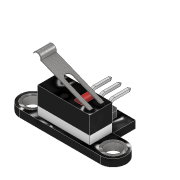
# Autodesk Inventor part: limit_switch
Saved by Autodesk Inventor 2022 (Build 260153000, 153)
## iProperties
Created: 2022-11-16
Part Number: limit_switch
Material: Generic
Document SubType Name: Modeling
Designer: ferna
Density: 1 g/cm^3
Appearance: Default
Author: ferna
Autodesk Inventor part; units mm, degrees
sketch "Sketch1" plane through (0, 0, 0) normal (0, 1, 0) x (-1, 0, 0)
  line L0 (0, 0) -> (14.5, 0)
  line L1 (14.5, 0) -> (14.5, -6)
  line L2 (14.5, -6) -> (0, -6)
  line L3 (0, -6) -> (0, 0)
  line L4 (0, 0) -> (14.5, 0)
  line L5 (14.5, 0) -> (14.5, 7)
  line L6 (14.5, 7) -> (0, 7)
  line L7 (0, 7) -> (0, 0)
  line L8 (14.5, 3.5) -> (18, 3.5)
  line L9 (0, 3.5) -> (-3.5, 3.5)
  circle A0 centre (18, 3.5) radius 3.5
  circle A1 centre (-3.5, 3.5) radius 3.5
  line L10 (18, 7) -> (14.5, 7)
  line L11 (18, 0) -> (14.5, 0)
  line L12 (0, 0) -> (-3.5, 0)
  line L13 (-3.5, 7) -> (0, 7)
  circle A2 centre (18, 3.5) radius 2
  circle A3 centre (-3.5, 3.5) radius 2
  dimension "d0" = 14.5
  dimension "d1" = 6
  dimension "d2" = 7
  dimension "d3" = 3.5
  dimension "d4" = 3.5
  dimension "d5" = 4
  constraints: 28 end point, 6 point on circle, 5 parallel, 4 centre point, 4 coincident, 4 horizontal, 2 midpoint, 2 perpendicular, 2 point on line, 2 tangent
  measures "d0" distance of L1.end L2.end
  measures "d1" distance of L0.end L1.end
  measures "d2" distance of L5.end L4.end
  measures "d3" distance of L8.start L8.end
  measures "d4" distance of L9.start L9.end
  measures "d5" diameter of A2
extrude "Extrusion1" add sketch "Sketch1" along normal blind 2
sketch "Sketch2" plane through (0, 2, 0) normal (0, 1, 0) x (1, 0, 0)
  line L0 (0, 0) -> (0, 6) projected
  line L1 (0, 0) -> (0, -3)
  line L2 (0, -3) -> (-7.25, -3)
  line L3 (-0.25, -6) -> (-14.25, -6)
  line L4 (-14.25, -6) -> (-14.25, 0)
  line L5 (-14.25, 0) -> (-0.25, 0)
  line L6 (-0.25, 0) -> (-0.25, -6)
  line L7 (-0.25, -6) -> (-14.25, 0) construction
  line L8 (-14.25, -6) -> (-0.25, 0) construction
  dimension "d8" = 3
  dimension "d9" = 7.25
  dimension "d10" = 14
  dimension "d11" = 6
  constraints: 16 end point, 2 midpoint, 2 parallel, 2 perpendicular, 1 horizontal, 1 vertical
  measures "d8" distance of L0.start L1.end
  measures "d9" distance of L1.end L2.end
  measures "d10" distance of L4.end L5.end
  measures "d11" distance of L3.end L4.end
extrude "Extrusion2" add sketch "Sketch2" along normal blind 7
ref_plane "Work Plane1" through (-14.25, 2, 5) normal (0, 0, 1) x (1, 0, 0)
sketch "Sketch3" plane through (-14.25, 2, 5) normal (0, 0, 1) x (1, 0, 0)
  line L0 (14, 7) -> (0, 7) projected
  line L1 (12.8898, 7) -> (0, 12.2078)
  line L2 (12.8898, 7) -> (26.7918, 7) construction
  line L3 (0, 12.2078) -> (0, 12.0078)
  line L4 (0, 12.0078) -> (12.3948, 7)
  line L5 (0, 12.0078) -> (13.3682, 12.0078) construction
  line L6 (12.3948, 7) -> (12.8898, 7)
  arc A0 (0, 12.2078) -> (-2.0675, 13.0431) centre (-1.0827, 12.5043) ccw
  line L7 (-2.0675, 13.0431) -> (-2.0675, 12.8431)
  arc A1 (-0.2257, 12.099) -> (-2.0675, 12.8431) centre (-1.1902, 12.3632) ccw
  line L8 (-0.2257, 12.099) -> (0, 12.0078)
  point P0 (14.25, -2)
  point P1 (-0.2257, 12.099)
  dimension "d15" = 158
  dimension "d16" = 0.2
  dimension "d17" = 22
  dimension "d18" = 0.2
  dimension "d19" = 1
  constraints: 16 end point, 4 point on circle, 3 horizontal, 3 point on line, 2 centre point, 2 equal length, 1 perpendicular, 1 vertical
  measures "d15" angle of L2 L1
  measures "d16" distance of L1.end L3.end
  measures "d17" angle of L4 L5
  measures "d18" distance of L7.start L7.end
  measures "d19" radius of A1
extrude "Extrusion3" add sketch "Sketch3" against normal blind 4
sketch "Sketch4" plane through (-18, 0, 7) normal (0, 0, 1) x (1, 0, 0)
  line L0 (0, 2) -> (-3.5, 2) projected
  line L1 (-3.5, 2) -> (26.8199, 2)
  line L2 (26.8199, 2) -> (26.8199, 16.7787)
  line L3 (26.8199, 16.7787) -> (-3.5, 16.7787)
  line L4 (-3.5, 16.7787) -> (-3.5, 2)
  point P0 (18, 0)
  constraints: 8 end point, 2 parallel, 1 horizontal, 1 perpendicular
split body "Split1" sketch "Sketch4" result two bodies curves L4 L1 L2 L3 first body at (-4.9167, 4.3333, 0.5)
sketch "Sketch5" plane through (-14.25, 9, 6) normal (0, 0, 1) x (1, 0, 0)
  line L0 (-3.2734, -4.7413) -> (21.2547, -4.7413)
  line L1 (21.2547, -4.7413) -> (21.2547, 8.151)
  line L2 (21.2547, 8.151) -> (-3.2734, 8.151)
  line L3 (-3.2734, 8.151) -> (-3.2734, -4.7413)
  point P0 (14.25, -9)
  constraints: 8 end point, 2 parallel, 1 horizontal, 1 perpendicular
split body "Split2" sketch "Sketch5" result two bodies bodies 2 curves L2 L3 L0 L1 first body at (-9.5833, 4.7587, 4)
sketch "Sketch6" plane through (-14.25, 9, 6) normal (0, 0, 1) x (1, 0, 0)
  line L0 (0, 0) -> (14, 0) projected
  line L1 (14, 0) -> (-4.9489, 0)
  line L2 (-4.9489, 0) -> (-4.9489, 7.5925)
  line L3 (-4.9489, 7.5925) -> (14, 7.5925)
  line L4 (14, 7.5925) -> (14, 0)
  point P0 (14.25, -9)
  constraints: 8 end point, 2 parallel, 1 horizontal, 1 perpendicular
split body "Split3" sketch "Sketch6" result two bodies bodies 4 curves L3 L4 L1 L2 first body at (-9.5833, 4.7587, 4)
sketch "Sketch7" plane through (0, 2, 0) normal (0, 1, 0) x (1, 0, 0)
  circle A0 centre (-18, -3.5) radius 2 projected
  circle A1 centre (3.5, -3.5) radius 2 projected
  circle A2 centre (-18, -3.5) radius 2.75
  circle A3 centre (3.5, -3.5) radius 2 projected
  circle A4 centre (3.5, -3.5) radius 2.75
  point P0 (0, 0)
  dimension "d22" = 5.5
  dimension "d23" = 5.5
  constraints: 2 centre point, 2 coincident
  measures "d22" diameter of A2
  measures "d23" diameter of A4
split body "Split4" sketch "Sketch7" result two bodies bodies 3 curves A2 first body at (-15.7573, 0.6667, 3.319)
sketch "Sketch8" plane through (0, 2, 0) normal (0, 1, 0) x (1, 0, 0)
  circle A0 centre (3.5, -3.5) radius 2 projected
  circle A1 centre (3.5, -3.5) radius 2.75
  point P0 (0, 0)
  dimension "d24" = 5.5
  constraints: 1 centre point, 1 coincident
  measures "d24" diameter of A1
split body "Split5" sketch "Sketch8" result two bodies bodies 9 curves A1 first body at (5.7427, 0.6667, 3.319)
ref_plane "Work Plane2" through (-14.25, 9, 3) normal (0, 0, 1) x (1, 0, 0)
sketch "Sketch9" plane through (-14.25, 9, 3) normal (0, 0, 1) x (1, 0, 0)
  line L0 (14, 0) -> (0, 0) projected
  arc A0 (10.6302, 0) -> (8.6302, 0) centre (9.6302, 0) ccw
  line L1 (8.6302, 0) -> (10.6302, 0)
  point P0 (14.25, -9)
  dimension "d26" = 1
  constraints: 2 end point, 2 point on circle, 2 point on line, 1 centre point, 1 collinear
  measures "d26" radius of A0
extrude "Extrusion4" add sketch "Sketch9" along normal mid plane 3.5 bodies 6
sketch "Sketch10" plane through (-14.25, 9, 3) normal (0, 0, 1) x (1, 0, 0)
  line L0 (14, 0) -> (0, 0) projected
  line L1 (11.2069, 0) -> (7.7665, 0)
  line L2 (7.7665, 0) -> (7.7665, 1.2584)
  line L3 (7.7665, 1.2584) -> (11.2069, 1.2584)
  line L4 (11.2069, 1.2584) -> (11.2069, 0)
  point P0 (14.25, -9)
  constraints: 8 end point, 2 parallel, 1 horizontal, 1 perpendicular, 1 point on line
split body "Split6" sketch "Sketch10" result two bodies bodies 6 curves L2 L3 L4 L1 first body at (-9.5833, 4.7587, 4)
sketch "Sketch11" plane through (-14.25, 14.2078, 5) normal (0.3746066, 0.9271839, 0) x (0.9271839, -0.3746066, 0)
  line L0 (13.9021, 0) -> (0, 0) projected
  line L1 (13.9021, 0) -> (13.9021, 1)
  line L2 (13.9021, 1) -> (5.9018, 1)
  line L3 (5.9018, 1) -> (5.9018, 3)
  line L4 (5.9018, 3) -> (13.9021, 3)
  line L5 (13.9021, 4) -> (13.9021, 0) projected
  line L6 (13.9021, 1) -> (13.9021, 3)
  circle A0 centre (5.9018, 2) radius 1
  point P0 (18.5347, 5)
  point P1 (5.9018, 1)
  dimension "d29" = 1
  dimension "d30" = 2
  constraints: 10 end point, 4 perpendicular, 1 midpoint, 1 point on line, 1 vertical, 3 other
  measures "d29" distance of L0.start L1.end
  measures "d30" distance of L2.end L3.end
extrude "Extrusion5" cut sketch "Sketch11" against normal blind 2 bodies 7
sketch "Sketch12" plane through (0, 2, 0) normal (0, 1, 0) x (1, 0, 0)
  line L0 (-10.8542, 2.9594) -> (-10.8542, 4.2294)
  line L1 (-10.8542, 4.2294) -> (-10.2192, 4.8644)
  line L2 (-10.2192, 4.8644) -> (-8.9492, 4.8644)
  line L3 (-9.9042, 3.8944) -> (-9.9042, 3.2544)
  line L4 (-9.9042, 3.2544) -> (-9.2642, 3.2544)
  line L5 (-9.2642, 3.8944) -> (-9.9042, 3.8944)
  line L6 (-9.2642, 3.2544) -> (-9.2642, 3.8944)
  line L7 (-8.9492, 4.8644) -> (-8.3142, 4.2294)
  line L8 (-8.3142, 4.2294) -> (-7.6792, 4.8644)
  line L9 (-7.6792, 4.8644) -> (-6.4092, 4.8644)
  line L10 (-6.4092, 4.8644) -> (-5.7742, 4.2294)
  line L11 (-5.7742, 4.2294) -> (-5.1392, 4.8644)
  line L12 (-5.1392, 4.8644) -> (-3.8692, 4.8644)
  line L13 (-3.8692, 4.8644) -> (-3.2342, 4.2294)
  line L14 (-3.2342, 2.9594) -> (-3.2342, 4.2294)
  line L15 (-3.2342, 2.9594) -> (-3.8692, 2.3244)
  line L16 (-5.1392, 2.3244) -> (-3.8692, 2.3244)
  line L17 (-5.1392, 2.3244) -> (-5.7742, 2.9594)
  line L18 (-5.7742, 2.9594) -> (-6.4092, 2.3244)
  line L19 (-7.6792, 2.3244) -> (-6.4092, 2.3244)
  line L20 (-7.6792, 2.3244) -> (-8.3142, 2.9594)
  line L21 (-8.3142, 2.9594) -> (-8.9492, 2.3244)
  line L22 (-10.2192, 2.3244) -> (-8.9492, 2.3244)
  line L23 (-10.2192, 2.3244) -> (-10.8542, 2.9594)
  line L24 (-7.3642, 3.8944) -> (-7.3642, 3.2544)
  line L25 (-6.7242, 3.8944) -> (-7.3642, 3.8944)
  line L26 (-7.3642, 3.2544) -> (-6.7242, 3.2544)
  line L27 (-6.7242, 3.2544) -> (-6.7242, 3.8944)
  line L28 (-4.8242, 3.8944) -> (-4.8242, 3.2544)
  line L29 (-4.1842, 3.8944) -> (-4.8242, 3.8944)
  line L30 (-4.1842, 3.2544) -> (-4.1842, 3.8944)
  line L31 (-4.8242, 3.2544) -> (-4.1842, 3.2544)
  point P0 (0, 0)
  constraints: 64 end point
extrude "Extrusion6" add sketch "Sketch12" along normal blind 1.5 separate body
sketch "Sketch13" plane through (0, 2, 0) normal (0, 1, 0) x (1, 0, 0)
  line L0 (-9.2642, 3.8944) -> (-9.2642, 3.2544) projected
  line L1 (-9.2642, 3.2544) -> (-9.9042, 3.2544) projected
  line L2 (-9.9042, 3.2544) -> (-9.9042, 3.8944) projected
  line L3 (-9.9042, 3.8944) -> (-9.2642, 3.8944) projected
  line L4 (-7.3642, 3.2544) -> (-7.3642, 3.8944) projected
  line L5 (-6.7242, 3.2544) -> (-7.3642, 3.2544) projected
  line L6 (-6.7242, 3.8944) -> (-6.7242, 3.2544) projected
  line L7 (-7.3642, 3.8944) -> (-6.7242, 3.8944) projected
  line L8 (-4.8242, 3.2544) -> (-4.8242, 3.8944) projected
  line L9 (-4.1842, 3.2544) -> (-4.8242, 3.2544) projected
  line L10 (-4.1842, 3.8944) -> (-4.1842, 3.2544) projected
  line L11 (-4.8242, 3.8944) -> (-4.1842, 3.8944) projected
  line L12 (-7.3642, 3.2544) -> (-7.3642, 3.8944) projected
  line L13 (-7.3642, 3.5744) -> (-7.0442, 3.5744)
  point P0 (0, 0)
  dimension "d35" = 0.32
  constraints: 2 end point, 1 horizontal, 1 midpoint
  measures "d35" distance of L13.start L13.end
ref_plane "Work Plane3" through (-7.0442, 2, -3.5744) normal (1, 0, 0) x (0, 0, -1)
sketch "Sketch14" plane through (-7.0442, 2, -3.5744) normal (1, 0, 0) x (0, 0, -1)
  line L0 (0, 0) -> (0, 2.5)
  line L1 (1, 3.5) -> (5, 3.5)
  arc A0 (1, 3.5) -> (0, 2.5) centre (1, 2.5) ccw
  point P0 (-3.5744, -2)
  point P1 (0, 3.5)
  dimension "d36" = 3.5
  dimension "d37" = 5
  dimension "d38" = 1
  constraints: 4 end point, 2 point on circle, 2 point on line, 2 tangent, 1 centre point, 1 perpendicular, 1 vertical
  measures "d36" distance of L0.start point (0, 3.5)
  measures "d37" distance of point (0, 3.5) L1.end
  measures "d38" radius of A0
sweep "Sweep1" add profiles "Sketch13" path "Sketch14" separate body
ref_plane "Work Plane4" through (-4.1842, 5.18, -9.0744) normal (0, 0, -1) x (-1, 0, 0)
sketch "Sketch15" plane through (-4.1842, 5.18, -9.0744) normal (0, 0, -1) x (-1, 0, 0)
  line L0 (5.72, 0.64) -> (5.08, 0.64) projected
  line L1 (5.72, 0.64) -> (5.72, 0.44)
  line L2 (5.72, 0) -> (5.72, 0.64) projected
  line L3 (5.72, 0.44) -> (5.52, 0.44)
  line L4 (5.08, 0.64) -> (5.08, 0) projected
  line L5 (5.52, 0.44) -> (3.18, 0.44)
  line L6 (3.18, -0.68) -> (3.18, 0.64) projected
  line L7 (3.18, 0.44) -> (2.98, 0.44)
  line L8 (2.98, 0.44) -> (0.64, 0.44)
  line L9 (0.64, 0) -> (0.64, 0.64) projected
  line L10 (0.64, 0.44) -> (0.44, 0.44)
  line L11 (0.44, 0.44) -> (0, 0.44)
  line L12 (0, 0.64) -> (0, 0) projected
  line L13 (5.52, 0.44) -> (5.28, 0.44)
  line L14 (5.28, 0.44) -> (5.28, 0.2)
  line L15 (5.28, 0.2) -> (5.52, 0.2)
  line L16 (5.52, 0.2) -> (5.52, 0.44)
  line L17 (2.98, 0.44) -> (2.74, 0.44)
  line L18 (2.74, 0.44) -> (2.74, 0.2)
  line L19 (2.74, 0.2) -> (2.98, 0.2)
  line L20 (2.98, 0.2) -> (2.98, 0.44)
  line L21 (0.44, 0.44) -> (0.2, 0.44)
  line L22 (0.2, 0.44) -> (0.2, 0.2)
  line L23 (0.2, 0.2) -> (0.44, 0.2)
  line L24 (0.44, 0.2) -> (0.44, 0.44)
  point P0 (-4.1842, -5.18)
  dimension "d42" = 0.2
  dimension "d43" = 0.2
  dimension "d44" = 0.2
  dimension "d45" = 0.2
  dimension "d46" = 0.24
  dimension "d47" = 0.24
  dimension "d48" = 0.24
  dimension "d49" = 0.24
  dimension "d50" = 0.24
  dimension "d51" = 0.24
  constraints: 38 end point, 9 point on line, 6 parallel, 4 perpendicular, 3 horizontal
  measures "d42" distance of L0.start L1.end
  measures "d43" distance of L1.end L3.end
  measures "d44" distance of L5.end L7.end
  measures "d45" distance of L8.end L10.end
  measures "d46" distance of L15.end L14.end
  measures "d47" distance of L14.end L13.end
  measures "d48" distance of L19.end L18.end
  measures "d49" distance of L18.end L17.end
  measures "d50" distance of L23.end L22.end
  measures "d51" distance of L22.end L21.end
loft "Loft1" add profiles "Sketch15" bodies 15 section 1 edges at (-9.9042, 5.5, -8.5744) (-9.5842, 5.82, -8.5744) (-9.2642, 5.5, -8.5744) (-9.5842, 5.18, -8.5744) contours L16 L15 L14 L5
sketch "Sketch16" plane through (-4.1842, 5.18, -9.0744) normal (0, 0, -1) x (-1, 0, 0)
  line L0 (3.18, 0.64) -> (2.98, 0.64)
  line L1 (3.18, 0.64) -> (2.54, 0.64) projected
  line L2 (2.98, 0.64) -> (2.98, 0.44)
  line L3 (2.98, 0.44) -> (2.74, 0.44)
  line L4 (2.74, 0.44) -> (2.74, 0.2)
  line L5 (2.74, 0.2) -> (2.98, 0.2)
  line L6 (2.98, 0.2) -> (2.98, 0.44)
  point P0 (-4.1842, -5.18)
  dimension "d56" = 0.2
  dimension "d57" = 0.2
  dimension "d58" = 0.24
  dimension "d59" = 0.24
  constraints: 12 end point, 2 parallel, 2 perpendicular, 1 horizontal, 1 point on line
  measures "d56" distance of L0.start L0.end
  measures "d57" distance of L0.end L2.end
  measures "d58" distance of L5.end L4.end
  measures "d59" distance of L4.end L3.end
loft "Loft2" add profiles "Sketch16" bodies 15 section 1 edges at (-6.7242, 5.5, -8.5744) (-7.0442, 5.18, -8.5744) (-7.3642, 5.5, -8.5744) (-7.0442, 5.82, -8.5744)
sketch "Sketch17" plane through (-4.1842, 5.18, -9.0744) normal (0, 0, -1) x (-1, 0, 0)
  line L0 (0.64, 0) -> (0.64, 0.64) projected
  line L1 (0.64, 0.64) -> (0.44, 0.64)
  line L2 (0.64, 0.64) -> (0, 0.64) projected
  line L3 (0.44, 0.64) -> (0.44, 0.44)
  line L4 (0.44, 0.44) -> (0.2, 0.44)
  line L5 (0.2, 0.44) -> (0.2, 0.2)
  line L6 (0.2, 0.2) -> (0.44, 0.2)
  line L7 (0.44, 0.2) -> (0.44, 0.44)
  point P0 (-4.1842, -5.18)
  dimension "d64" = 0.2
  dimension "d65" = 0.2
  dimension "d66" = 0.24
  dimension "d67" = 0.24
  constraints: 12 end point, 2 parallel, 2 perpendicular, 1 horizontal, 1 point on line
  measures "d64" distance of L0.end L1.end
  measures "d65" distance of L1.end L3.end
  measures "d66" distance of L6.end L5.end
  measures "d67" distance of L5.end L4.end
loft "Loft3" add profiles "Sketch17" bodies 15 section 1 edges at (-4.1842, 5.5, -8.5744) (-4.5042, 5.18, -8.5744) (-4.8242, 5.5, -8.5744) (-4.5042, 5.82, -8.5744)
body "Solid14"
body "Solid15"
body "Solid5"
body "Solid7"
body "Solid8"
body "Solid10"
body "Solid11"
body "Solid12"
body "Solid13"
